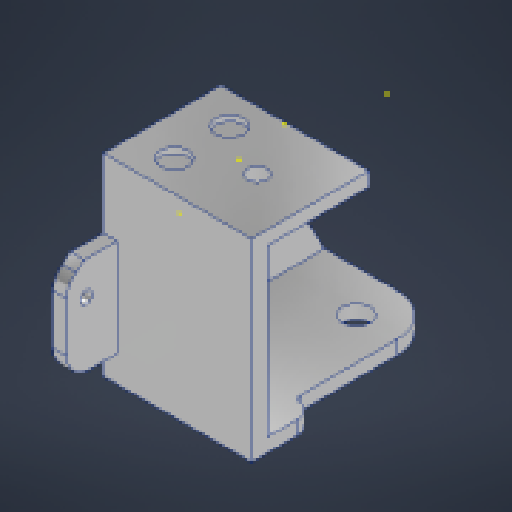
# Autodesk Inventor part: DC23[R][F][2]
Saved by Autodesk Inventor 2024 (Build 280153000, 153)
## iProperties
Created: 2022-10-25
Part Number: DC23[R][F][2]
Material: Aluminio 6061
Document SubType Name: Modeling
Designer: juanr
Density: 2.7 g/cm^3
Appearance: Aluminio - Plano
Author: juanr
Autodesk Inventor part; units mm, degrees
ref_plane "YZ Plane" through (0, 0, 0) normal (1, 0, 0) x (0, 1, 0)
ref_plane "XZ Plane" through (0, 0, 0) normal (0, 1, 0) x (-1, 0, 0)
ref_plane "XY Plane" through (0, 0, 0) normal (0, 0, 1) x (1, 0, 0)
sketch "Sketch1" plane through (0, 0, 0) normal (0, 1, 0) x (-1, 0, 0)
  line L0 (0, -25.5) -> (-34.15, -25.5)
  line L1 (-34.15, -25.5) -> (-34.15, 0)
  line L2 (-34.15, 0) -> (-34.15, 25.5)
  line L3 (-34.15, 25.5) -> (0, 25.5)
  line L4 (0, 25.5) -> (34.15, 25.5)
  line L5 (34.15, 25.5) -> (34.15, 0)
  line L6 (34.15, 0) -> (34.15, -25.5)
  line L7 (34.15, -25.5) -> (0, -25.5)
  point P0 (0, 0)
  constraints: 16 end point, 3 perpendicular, 2 point on line, 1 horizontal, 1 vertical
extrude "Extrusion1" add sketch "Sketch1" along normal blind 7
sketch "Sketch3" plane through (-34.15, 0, 25.5) normal (0, 0, 1) x (1, 0, 0)
  line L0 (0, 0) -> (0, -78.85)
  point P0 (34.15, 0)
  dimension "d7" = 78.85
  constraints: 2 end point, 1 vertical
  measures "d7" distance of L0.start L0.end
sketch "Sketch4" plane through (-34.15, 0, -25.5) normal (-1, 0, 0) x (0, 0, 1)
  line L0 (51, 0) -> (51, -78.85)
  line L1 (51, -78.85) -> (-39, -78.85)
  line L2 (-39, -78.85) -> (-39, -71.85)
  line L3 (0, 0) -> (-39, -71.85)
  line L4 (0, 0) -> (51, 0)
  point P0 (25.5, 0)
  dimension "d10" = 90
  dimension "d11" = 7
  constraints: 10 end point, 2 horizontal, 2 vertical
  measures "d10" distance of L0.end L1.end
  measures "d11" distance of L1.end L2.end
extrude "Extrusion2" add sketch "Sketch4" against normal blind 7
sketch "Sketch6" plane through (0, 7, 0) normal (0, 1, 0) x (1, 0, 0)
  line L0 (34.15, -25.5) -> (34.15, 25.5) projected
  line L1 (34.15, 25.5) -> (34.15, 0)
  line L2 (-34.15, 25.5) -> (-34.15, -25.5) projected
  circle A0 centre (8.15, 0) radius 5
  point P0 (0, 0)
  dimension "d20" = 10
  constraints: 2 end point, 1 centre point, 1 midpoint
  measures "d20" diameter of A0
extrude "Extrusion4" cut sketch "Sketch6" against normal blind 10
sketch "Sketch7" plane through (-27.15, 0, -25.5) normal (1, 0, 0) x (0, 0, -1)
  line L0 (-51, -78.85) -> (39, -78.85) projected
  line L1 (-51, -78.85) -> (39, -78.85)
  line L2 (39, -78.85) -> (39, -71.85) projected
  line L3 (39, -78.85) -> (39, -71.85)
  line L4 (39, -71.85) -> (-51, -71.85)
  line L5 (-51, 0) -> (-51, -78.85) projected
  line L6 (-51, -78.85) -> (-51, -71.85)
  point P0 (-25.5, 0)
  constraints: 8 end point, 2 perpendicular, 1 collinear, 1 horizontal, 1 point on line
sketch "Sketch8" plane through (0, 0, 0) normal (0, -1, 0) x (1, 0, 0)
  circle A0 centre (8.15, 0) radius 5 projected
  line L0 (8.15, 18.5) -> (34.15, 18.5)
  line L1 (34.15, 25.5) -> (34.15, -25.5) projected
  line L2 (8.15, 25.5) -> (34.15, 25.5)
  line L3 (8.15, 25.5) -> (-27.15, 25.5)
  line L4 (-27.15, 25.5) -> (-27.15, -25.5) projected
  line L5 (8.15, 18.5) -> (-27.15, 18.5)
  line L6 (34.15, 25.5) -> (34.15, 18.5)
  line L7 (-27.15, 25.5) -> (-27.15, 18.5)
  point P0 (0, 0)
  constraints: 12 end point, 2 collinear, 2 point on line, 1 horizontal, 1 parallel
extrude "Extrusion6" add sketch "Sketch7" along normal blind 58.5
extrude "Extrusion7" add sketch "Sketch8" along normal blind 78.75 contours L5 L4 L3 L2 L1 L0
sketch "Sketch9" plane through (31.35, 0, -25.5) normal (1, 0, 0) x (0, 0, -1)
  line L0 (-51, -78.75) -> (-51, 7) projected
  line L1 (-44, 0) -> (-44, -71.85) projected
  line L2 (-51, -78.75) -> (-44, -78.75)
  line L3 (-44, -78.75) -> (-44, -71.85)
  line L4 (-44, -71.85) -> (-51, -71.85)
  line L5 (-51, -71.85) -> (-51, -78.75)
  point P0 (-25.5, 0)
  constraints: 8 end point, 2 parallel, 1 horizontal, 1 perpendicular
extrude "Extrusion8" cut sketch "Sketch9" along normal blind 10
sketch "Sketch10" plane through (0, 7, 0) normal (0, 1, 0) x (1, 0, 0)
  point P0 (0, 0)
sketch "Boceto11" plane through (-34.15, -78.85, -64.5) normal (0, -1, 0) x (1, 0, 0)
  line L0 (72.0718, 89.9914) -> (72.0718, 37.9883)
  line L1 (72.0718, 37.9883) -> (65.5278, 37.9883)
  line L2 (65.5278, 37.9883) -> (65.5278, 89.9914)
  line L3 (72.0718, 89.9914) -> (72.0718, 92.1751)
  line L4 (72.0718, 92.1751) -> (65.5278, 92.1751)
  line L5 (65.5278, 92.1751) -> (65.5278, 89.9914)
  point P0 (34.15, 64.5)
  constraints: 12 end point, 2 perpendicular, 1 parallel, 1 vertical
extrude "Extrusión9" cut sketch "Boceto11" against normal blind 1000
sketch "Boceto18" plane through (-34.15, -78.85, 25.5) normal (0, 0, 1) x (1, 0, 0)
  point P0 (34.15, 78.85)
sketch "Boceto23" plane through (-27.15, 0, -25.5) normal (0, 0.4770514, -0.8788754) x (-1, 0, 0)
  point P0 (-27.15, 12.1648)
sketch "Boceto24" plane through (-27.15, 0, -25.5) normal (0, 0, -1) x (-1, 0, 0)
  line L0 (7, -71.85) -> (7, -78.85) projected
  line L1 (7, -78.35) -> (7, -78.85)
  line L2 (7, -78.85) -> (-58.5, -78.85) projected
  line L3 (-58.5, -78.85) -> (-58.5, -77.85)
  line L4 (-58.5, -71.85) -> (-58.5, -78.85) projected
  line L5 (-58.5, -77.85) -> (6, -77.85)
  line L6 (7, -77.85) -> (7, -78.85)
  line L7 (7, -78.85) -> (-58.8392, -78.85)
  line L8 (-58.5278, 7) -> (7, 7) projected
  line L9 (7, -78.85) -> (7, 7)
  line L10 (7, 7) -> (6, 7)
  line L11 (6, 6) -> (6, -77.85)
  line L12 (-58.5278, -71.85) -> (-58.5278, 7) projected
  line L13 (-58.5278, 7) -> (-58.5278, 6)
  line L14 (-58.5278, 6) -> (6, 6)
  line L15 (7, 0) -> (7, 7) projected
  line L16 (7, 6) -> (7, 7)
  line L17 (7, 7) -> (-58.5278, 7)
  point P0 (-27.15, 0)
  dimension "d65" = 1
  dimension "d66" = 1
  dimension "d67" = 1
  constraints: 24 end point, 7 perpendicular, 5 point on line, 1 collinear, 1 horizontal, 1 vertical
  measures "d65" distance of L2.end L3.end
  measures "d66" distance of L8.end L10.end
  measures "d67" distance of L8.start L13.end
extrude "Extrusión19" cut sketch "Boceto24" along normal mid plane 1000
sketch "Boceto25" plane through (31.35, -71.85, -64.5) normal (0, 0, -1) x (-1, 0, 0)
  point P0 (31.35, 71.85)
sketch "Boceto27" plane through (31.3778, 0, -25.5) normal (0, 0, -1) x (-1, 0, 0)
  line L0 (0, -71.85) -> (0, 6) projected
  line L1 (0, 6) -> (0.228, 6)
  line L2 (0, 6) -> (64.5278, 6) projected
  line L3 (0.228, 6) -> (0.228, -77.85)
  line L4 (0.0278, -77.85) -> (64.5278, -77.85) projected
  line L5 (0.0278, -71.85) -> (0.0278, -77.85) projected
  line L6 (0.228, -77.85) -> (0.0278, -77.85)
  line L7 (0.0278, -77.85) -> (0, 6)
  line L8 (0, 6) -> (0, -77.85)
  line L9 (0, -77.85) -> (0.0278, -77.85)
  point P0 (31.3778, 0)
  dimension "d73" = 0.228
  constraints: 12 end point, 3 perpendicular, 3 point on line, 1 horizontal
  measures "d73" distance of L0.end L1.end
extrude "Extrusión21" cut sketch "Boceto27" along normal mid plane 1000
sketch "Boceto28" plane through (-33.15, 0, -25.5) normal (-1, 0, 0) x (0, 0, 1)
  point P0 (25.5, 0)
sketch "Boceto30" plane through (-33.15, 0, -25.5) normal (-1, 0, 0) x (0, 0, 1)
  point P0 (25.5, 0)
sketch "Boceto31" plane through (-33.15, 0, -25.5) normal (-1, 0, 0) x (0, 0, 1)
  circle A0 centre (64.38, -38.5153) radius 2.6
  point P0 (25.5, 0)
  point P1 (64.38, -49.4573)
  constraints: 1 centre point
sketch "Boceto32" plane through (-27.15, -71.85, 18.5) normal (0, 1, 0) x (1, 0, 0)
  circle A0 centre (47, 71.5) radius 5 projected
  circle A1 centre (47, 71.5) radius 5
  line L0 (52, 71.5) -> (58.2998, 71.5)
  line L1 (67, 83) -> (67, -7)
  line L2 (58.2998, -7) -> (-6, -7) projected
  line L3 (67, -7) -> (58.2998, -7)
  line L4 (58.2998, -7) -> (58.2998, 83)
  line L5 (47, 76.5) -> (47, 83)
  line L6 (-6, 83) -> (0, 83) projected
  line L7 (-6, 83) -> (-6, 91.5)
  line L8 (-6, 91.5) -> (67, 91.5)
  line L9 (67, 91.5) -> (67, 83)
  line L10 (-6, 83) -> (58.2998, 83)
  point P0 (27.15, 18.5)
  constraints: 18 end point, 2 perpendicular, 2 point on circle, 2 point on line, 2 vertical, 1 centre point, 1 coincident, 1 collinear, 1 horizontal
extrude "Extrusión23" add sketch "Boceto32" against normal blind 6 contours L4 L10 L6 L7 L8 L9 L1 L3
sketch "Boceto33" plane through (-33.15, -77.85, 25.5) normal (-1, 0, 0) x (0, 0, 1)
  line L0 (0, 83.85) -> (0, 0) projected
  line L1 (0, 74.4354) -> (10.1255, 74.4354)
  line L2 (10.1255, 74.4354) -> (10.1255, 56.6115)
  line L3 (10.9445, 54.9975) -> (18.0243, 49.8171)
  line L4 (18.8039, 48.5979) -> (20.1084, 42.1205)
  line L5 (0, 11.6181) -> (18.1478, 11.6181)
  line L6 (20.1478, 13.6181) -> (20.1478, 41.7256)
  arc A0 (10.1255, 56.6115) -> (10.9445, 54.9975) centre (12.1255, 56.6115) ccw
  arc A1 (18.8039, 48.5979) -> (18.0243, 49.8171) centre (16.8433, 48.203) ccw
  arc A2 (20.1478, 41.7256) -> (20.1084, 42.1205) centre (18.1478, 41.7256) ccw
  arc A3 (18.1478, 11.6181) -> (20.1478, 13.6181) centre (18.1478, 13.6181) ccw
  point P0 (-25.5, 77.85)
  dimension "d91" = 2
  constraints: 12 end point, 8 point on circle, 8 tangent, 4 centre point, 3 equal radius, 2 horizontal, 2 perpendicular, 2 point on line
  measures "d91" radius of A0
extrude "Extrusión24" add sketch "Boceto33" against normal blind 6
extrude "Extrusión25" cut sketch "Boceto31" against normal blind 6
sketch "Boceto34" plane through (-27.15, -77.85, 25.5) normal (1, 0, 0) x (0, 0, -1)
  line L0 (-18.1478, 11.6181) -> (-21.8775, 11.6181)
  line L1 (-21.8775, 11.6181) -> (-21.8775, 48.067)
  line L2 (-21.8775, 48.067) -> (-10.1255, 56.8358)
  line L3 (-10.1255, 74.4354) -> (-10.1255, 56.6115) projected
  line L4 (-10.1255, 56.8358) -> (-10.1255, 48.9642)
  line L5 (-10.1255, 48.9642) -> (-16.6729, 42.1735)
  line L6 (-16.6729, 42.1735) -> (-18.1478, 11.6181)
  point P0 (25.5, 77.85)
  constraints: 12 end point, 1 horizontal, 1 perpendicular, 1 point on line, 1 vertical
extrude "Extrusión26" add sketch "Boceto34" against normal blind 6
fillet "Empalme5" radius 10 3 edges at (-30.15, -21.0142, 35.6255) (-30.15, -29.783, 47.3775) (-30.15, -66.2319, 47.3775)
sketch "Boceto37" plane through (-33.15, 6, 25.5) normal (0, 1, 0) x (1, 0, 0)
  circle A0 centre (41.3, 25.5) radius 6 projected
  line L0 (41.3, 25.5) -> (17.3, 25.5)
  line L1 (17.3, 25.5) -> (17.3, 13.5)
  line L2 (17.3, 13.5) -> (17.3, 37.5)
  circle A1 centre (17.3, 13.5) radius 6
  circle A2 centre (17.3, 37.5) radius 6
  point P0 (33.15, 25.5)
  dimension "d106" = 24
  dimension "d107" = 12
  dimension "d108" = 24
  dimension "d109" = 12
  dimension "d110" = 12
  constraints: 6 end point, 2 centre point, 2 coincident, 1 horizontal, 1 perpendicular, 1 point on line
  measures "d106" distance of L0.start L0.end
  measures "d107" distance of L0.end L1.end
  measures "d108" distance of L1.end L2.end
  measures "d109" diameter of A1
  measures "d110" diameter of A2
extrude "Extrusión29" cut sketch "Boceto37" against normal blind 2.5 contours A1 | A2
sketch "Boceto39" plane through (-27.15, -71.85, 18.5) normal (0, 1, 0) x (1, 0, 0)
  line L0 (58.2998, -7) -> (58.2998, 0)
  line L1 (58.2998, 44) -> (58.2998, 91.5)
  line L2 (-6, 91.5) -> (67, 91.5) projected
  line L3 (0, 0) -> (58.2998, 0) projected
  line L4 (58.2998, 0) -> (58.2998, -7) projected
  line L5 (58.2998, -7) -> (67, -7) projected
  line L6 (58.2998, -7) -> (67, -7)
  line L7 (67, 91.5) -> (-6, 91.5) projected
  line L8 (67, -7) -> (67, 91.5)
  line L9 (67, 91.5) -> (58.2998, 91.5)
  line L10 (58.2998, 0) -> (58.2998, 44)
  point P0 (27.15, 18.5)
  constraints: 12 end point, 3 collinear, 2 point on line, 1 perpendicular, 1 vertical
extrude "Extrusión31" cut sketch "Boceto39" against normal blind 10
sketch "Boceto41" plane through (-27.15, -71.85, 18.5) normal (0, 1, 0) x (1, 0, 0)
  line L0 (58.2998, 91.5) -> (58.2998, -7) projected
  line L1 (58.2998, 91.5) -> (31.7998, 91.5)
  line L2 (31.7998, 91.5) -> (31.7998, 65)
  line L3 (31.7998, 65) -> (58.2998, 65)
  line L4 (58.2998, 65) -> (58.2998, 91.5)
  circle A0 centre (31.7998, 65) radius 6
  point P0 (27.15, 18.5)
  dimension "d124" = 26.5
  dimension "d125" = 26.5
  dimension "d126" = 12
  constraints: 8 end point, 2 parallel, 1 centre point, 1 coincident, 1 horizontal, 1 perpendicular
  measures "d124" distance of L3.end L2.end
  measures "d125" distance of L2.end L1.end
  measures "d126" diameter of A0
extrude "Extrusión32" cut sketch "Boceto41" against normal blind 10 contours A0 L2 L3 | L3 L2 A0
sketch "Sketch42" plane through (-27.15, -71.85, 18.5) normal (0, 1, 0) x (1, 0, 0)
  circle A0 centre (31.7998, 65) radius 6 projected
  line L0 (31.7998, 71) -> (31.7998, 65)
  circle A1 centre (31.7998, 65) radius 18
  line L1 (0, 0) -> (0, 83) projected
  line L2 (0, 83) -> (31.7998, 83)
  line L3 (58.2998, 91.5) -> (-6, 91.5) projected
  line L4 (49.7998, 65) -> (49.7998, 0)
  line L5 (58.2998, 0) -> (0, 0) projected
  line L6 (0, 0) -> (58.2998, 0) projected
  line L7 (49.7998, 0) -> (58.2998, 0)
  line L8 (58.2998, 91.5) -> (58.2998, -7) projected
  line L9 (58.2998, 0) -> (58.2998, 91.5)
  line L10 (0, 83) -> (0, 44) projected
  line L11 (0, 83) -> (-6, 83)
  line L12 (-6, 91.5) -> (-6, 83) projected
  line L13 (-6, 83) -> (-6, 91.5)
  line L14 (58.2998, 91.5) -> (58.2998, 0) projected
  line L15 (-6, 91.5) -> (58.2998, 91.5)
  point P0 (27.15, 18.5)
  point P1 (58.2998, -7)
  dimension "d129" = 36
  constraints: 16 end point, 3 vertical, 2 collinear, 2 point on circle, 1 centre point, 1 coincident, 1 horizontal, 1 parallel, 1 perpendicular, 1 point on line, 1 vertical alignment, 2 other
  measures "d129" diameter of A1
extrude "Extrusion33" cut sketch "Sketch42" against normal blind 10 contours A1 L2 L11 L12 L3 L8 L5 L4
sketch "Sketch43" plane through (-27.15, -71.85, 18.5) normal (0, 0, -1) x (-1, 0, 0)
  line L0 (6, -6) -> (-58.2998, -6) projected
  line L1 (0, 0) -> (-49.7998, 0) projected
  line L2 (-58.2998, -6) -> (-49.7998, -6)
  line L3 (-49.7998, -6) -> (-49.7998, 0)
  line L4 (-49.7998, 0) -> (-58.2998, 0)
  line L5 (-58.2998, 0) -> (-58.2998, -6)
  point P0 (-27.15, 71.85)
  constraints: 8 end point, 2 parallel, 1 horizontal, 1 perpendicular
extrude "Extrusion34" add sketch "Sketch43" along normal blind 20
fillet "Fillet7" radius 7 1 edges at (31.1498, -74.85, -1.5)
fillet "Fillet8" radius 2 1 edges at (22.6498, -74.85, -1.5)
sketch "Sketch44" plane through (-33.15, 0, -25.5) normal (-1, 0, 0) x (0, 0, 1)
  line L0 (68.8577, -26.7837) -> (65.1452, -24.0136) projected
  line L1 (61.1255, -3.4146) -> (51, -3.4146) projected
  line L2 (65.1452, -24.0136) -> (51, -24.0136)
  line L3 (51, -24.0136) -> (51, -3.4146)
  line L4 (51, -3.4146) -> (65.1452, -3.4146)
  line L5 (65.1452, -3.4146) -> (65.1452, -24.0136)
  point P0 (25.5, 0)
  constraints: 8 end point, 2 parallel, 1 horizontal, 1 perpendicular
extrude "Extrusion35" cut sketch "Sketch44" against normal blind 20
sketch "Sketch45" plane through (-33.15, 6, 25.5) normal (0, 1, 0) x (1, 0, 0)
  circle A0 centre (41.3, 25.5) radius 5 projected
  circle A1 centre (41.3, 25.5) radius 4.25
  circle A2 centre (41.3, 25.5) radius 5
  point P0 (33.15, 25.5)
  dimension "d138" = 8.5
  constraints: 2 centre point, 2 coincident, 1 concentric
  measures "d138" diameter of A1
extrude "Extrusion36" add sketch "Sketch45" against normal blind 6
sketch "Sketch46" plane through (-33.15, 0, -25.5) normal (-1, 0, 0) x (0, 0, 1)
  point P0 (25.5, 0)
sketch "Sketch47" plane through (-33.15, 0, -25.5) normal (-1, 0, 0) x (0, 0, 1)
  line L0 (-44.1201, -43.7798) -> (-41.0263, -28.4947)
  line L1 (-39, -71.85) -> (0, 0) projected
  line L2 (-41.0263, -28.4947) -> (0, 0)
  line L3 (0, 0) -> (-39, -71.85)
  line L4 (-44.1201, -43.7798) -> (-44.1201, -71.85)
  line L5 (-44.1201, -71.85) -> (-39, -71.85)
  point P0 (25.5, 0)
  constraints: 10 end point, 1 collinear, 1 perpendicular, 1 vertical
extrude "Extrusion37" add sketch "Sketch47" against normal blind 6
sketch "Sketch48" plane through (-33.15, 6, -25.5) normal (-1, 0, 0) x (0, 0, 1)
  point P0 (25.5, -6)
sketch "Sketch49" plane through (-33.15, 6, -25.5) normal (-1, 0, 0) x (0, 0, 1)
  point P0 (25.5, -6)
sketch "Sketch50" plane through (-33.15, 6, -25.5) normal (-1, 0, 0) x (0, 0, 1)
  line L0 (-44.1201, -49.7798) -> (-41.0263, -34.4947) projected
  line L1 (-41.0263, -34.4947) -> (-46.4891, -61.4839)
  line L2 (-39, -83.85) -> (51, -83.85) projected
  line L3 (-39, -83.85) -> (-46.4891, -83.85)
  line L4 (-46.4891, -83.85) -> (-46.4891, -61.4839)
  line L5 (-41.0263, -34.4947) -> (-39, -69.2782)
  line L6 (-39, -69.2782) -> (-39, -83.85)
  point P0 (25.5, -6)
  constraints: 10 end point, 1 collinear, 1 horizontal, 1 perpendicular, 1 vertical
extrude "Extrusion38" add sketch "Sketch50" against normal blind 6
sketch "Sketch51" plane through (-33.15, 6, -25.5) normal (-1, 0, 0) x (0, 0, 1)
  line L0 (-41.0263, -34.4947) -> (-46.4891, -61.4839) projected
  line L1 (-41.0263, -34.4947) -> (-46.4891, -61.4839)
  line L2 (-46.4891, -61.4839) -> (-15.8808, -61.4839)
  line L3 (-41.0263, -34.4947) -> (-15.8808, -34.4947)
  line L4 (-15.8808, -34.4947) -> (-15.8808, -61.4839)
  point P0 (25.5, -6)
  constraints: 8 end point, 2 horizontal, 1 collinear, 1 perpendicular
extrude "Extrusion39" add sketch "Sketch51" along normal blind 9
sketch "Sketch52" plane through (-33.15, -55.4839, -71.9891) normal (0, -1, 0) x (1, 0, 0)
  line L0 (-9, 30.6084) -> (0, 53.8004)
  line L1 (0, 0) -> (0, 97.4891) projected
  line L2 (0, 30.6084) -> (0, 53.8004)
  line L3 (0, 30.6084) -> (-9, 30.6084)
  point P0 (33.15, 71.9891)
  constraints: 6 end point, 2 point on line, 1 collinear, 1 perpendicular
extrude "Extrusion40" add sketch "Sketch52" against normal blind 26.989
sketch "Sketch53" plane through (-33.15, -55.4839, -18.1887) normal (-0.9322642, 0, 0.3617781) x (0.3617781, 0, 0.9322642)
  point P0 (28.9496, 55.4839)
sketch "Sketch54" plane through (-33.15, 6, -25.5) normal (-1, 0, 0) x (0, 0, 1)
  line L0 (51, -72.2319) -> (51, -83.85) projected
  line L1 (51, -83.85) -> (86.3988, -83.85)
  line L2 (86.3988, -83.85) -> (86.3988, -18.2813)
  line L3 (86.3988, -18.2813) -> (51, -18.2813)
  line L4 (51, -18.2813) -> (51, -83.85)
  point P0 (25.5, -6)
  constraints: 8 end point, 2 parallel, 1 horizontal, 1 perpendicular
extrude "Extrusion41" cut sketch "Sketch54" against normal blind 26.989
body "Solid1"
